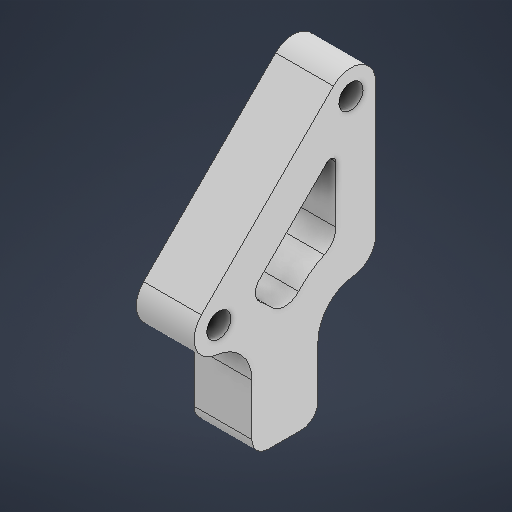
# Autodesk Inventor part: MOGO Mech
Saved by Autodesk Inventor 2025.1 (Build 291241000, 241)
## iProperties
Created: 2024-11-22
Part Number: MOGO Mech
Material: Generic
Document SubType Name: Modeling
Designer: Juanl
Density: 1 g/cm^3
Appearance: Default
Mass: 11.7203 g
Surface Area: 40.8724 cm^2
Volume: 11.7203 cm^3
Author: Juanl
Autodesk Inventor part; units mm, degrees
ref_plane "YZ Plane" through (0, 0, 0) normal (1, 0, 0) x (0, 1, 0)
ref_plane "XZ Plane" through (0, 0, 0) normal (0, 1, 0) x (-1, 0, 0)
ref_plane "XY Plane" through (0, 0, 0) normal (0, 0, 1) x (1, 0, 0)
sketch "Sketch1" plane through (0, 0, 0) normal (1, 0, 0) x (0, 1, 0)
  line L0 (-12.6683, 12.8416) -> (-12.6683, 0.1416)
  line L1 (-12.6683, 0.1416) -> (-12.6683, -12.5584)
  line L2 (-12.6683, -12.5584) -> (0.0318, -12.5584)
  line L3 (0.0318, -12.5584) -> (12.7318, -12.5584)
  circle A0 centre (-12.6683, 12.8416) radius 2.3241
  circle A1 centre (12.7318, -12.5584) radius 2.3241
  line L4 (-12.6683, 12.8416) -> (-12.6683, -12.5584) construction
  line L5 (-17.4308, 12.8416) -> (-17.4308, -12.5584)
  line L6 (-7.9058, -12.5584) -> (-7.9058, 12.8416)
  arc A2 (-7.9058, 12.8416) -> (-17.4308, 12.8416) centre (-12.6683, 12.8416) ccw
  arc A3 (-17.4308, -12.5584) -> (-7.9058, -12.5584) centre (-12.6683, -12.5584) ccw
  line L7 (12.7318, -12.5584) -> (-12.6683, -12.5584) construction
  line L8 (12.7318, -7.7959) -> (-12.6683, -7.7959)
  line L9 (-12.6683, -17.3209) -> (12.7318, -17.3209)
  arc A4 (12.7318, -17.3209) -> (12.7318, -7.7959) centre (12.7318, -12.5584) ccw
  arc A5 (-12.6683, -7.7959) -> (-12.6683, -17.3209) centre (-12.6683, -12.5584) ccw
  line L10 (-12.6683, 0.1416) -> (-38.0683, 0.1416)
  arc A6 (-7.9058, 4.3417) -> (-7.9058, -4.0585) centre (-12.6683, 0.1416) ccw
  line L11 (-12.6683, 6.4916) -> (-34.8933, 6.4916)
  line L12 (-38.0683, 3.3166) -> (-38.0683, -3.0334)
  line L13 (-34.8933, -6.2084) -> (-12.6683, -6.2084)
  arc A7 (-34.8933, 6.4916) -> (-38.0683, 3.3166) centre (-34.8933, 3.3166) ccw
  arc A8 (-38.0683, -3.0334) -> (-34.8933, -6.2084) centre (-34.8933, -3.0334) ccw
  point P0 (0, 0)
  point P1 (0.0317, -12.5584)
  point P2 (-7.9058, -7.7959)
  point P3 (-17.4308, -6.2084)
  point P4 (-17.4308, 6.4916)
  dimension "d1" = 4.6482
  dimension "d2" = 4.6482
  dimension "d3" = 9.525
  dimension "d7" = 25.4
  dimension "d8" = 12.7
  dimension "d9" = 3.175
  constraints: 32 end point, 16 point on circle, 13 tangent, 9 centre point, 5 point on line, 3 coincident, 3 perpendicular, 2 collinear, 2 parallel, 2 vertical, 1 concentric, 1 equal radius, 1 horizontal, 1 midpoint
  measures "d1" diameter of A0
  measures "d2" diameter of A1
  measures "d3" diameter of A3
  measures "d7" distance of L0.end L10.end
  measures "d8" diameter of A6
  measures "d9" radius of A7
extrude "Extrusion1" add sketch "Sketch1" along normal blind 11.1125
fillet "Fillet1" radius 7.62 1 edges at (5.5563, -17.4308, -6.2084)
sketch "Sketch3" plane through (11.1125, 0, 0) normal (1, 0, 0) x (0, 0, -1)
  arc A0 (-12.8416, -7.9058) -> (-12.8416, -17.4308) centre (-12.8416, -12.6683) ccw projected
  line L0 (-12.8416, -17.4308) -> (-6.4916, -17.4308) projected
  line L1 (-6.4916, -17.4308) -> (-6.4916, -34.8933) projected
  arc A1 (-6.4916, -34.8933) -> (-3.3166, -38.0683) centre (-3.3166, -34.8933) ccw projected
  line L2 (-3.3166, -38.0683) -> (3.0334, -38.0683) projected
  arc A2 (3.0334, -38.0683) -> (6.2084, -34.8933) centre (3.0334, -34.8933) ccw projected
  line L3 (6.2084, -34.8933) -> (6.2084, -24.9854) projected
  arc A3 (13.0468, -17.4056) -> (6.2084, -24.9854) centre (13.8284, -24.9854) ccw projected
  arc A4 (13.0468, -17.4056) -> (17.3209, -12.6683) centre (12.5584, -12.6683) ccw projected
  line L4 (17.3209, -12.6683) -> (17.3209, 12.7318) projected
  arc A5 (17.3209, 12.7318) -> (7.7959, 12.7318) centre (12.5584, 12.7318) ccw projected
  line L5 (7.7959, 12.7318) -> (7.7959, -7.9058) projected
  line L6 (7.7959, -7.9058) -> (-12.8416, -7.9058) projected
  circle A6 centre (-12.8416, -12.6683) radius 2.3241 projected
  circle A7 centre (12.5584, 12.7318) radius 2.3241 projected
  line L7 (-16.2092, -9.3007) -> (9.1908, 16.0993)
  arc A8 (-12.8416, -7.9058) -> (-12.8416, -17.4308) centre (-12.8416, -12.6683) ccw projected
  point P0 (0, 0)
  constraints: 2 end point, 2 point on circle, 2 tangent
extrude "Extrusion2" add sketch "Sketch3" against normal up to surface (11.1125 mm away) contours A0 L7 A5 L5 L6
fillet "Fillet2" radius 7.62 1 edges at (5.5563, -17.4308, 6.4916)
sketch "Sketch4" plane through (11.1125, 0, 0) normal (1, 0, 0) x (0, 0, -1)
  arc A0 (-16.2092, -9.3007) -> (-13.3301, -17.4056) centre (-12.8416, -12.6683) ccw projected
  arc A1 (-6.4916, -24.9854) -> (-13.3301, -17.4056) centre (-14.1116, -24.9854) ccw projected
  line L0 (-6.4916, -24.9854) -> (-6.4916, -34.8933) projected
  arc A2 (-6.4916, -34.8933) -> (-3.3166, -38.0683) centre (-3.3166, -34.8933) ccw projected
  line L1 (-3.3166, -38.0683) -> (3.0334, -38.0683) projected
  arc A3 (3.0334, -38.0683) -> (6.2084, -34.8933) centre (3.0334, -34.8933) ccw projected
  line L2 (6.2084, -34.8933) -> (6.2084, -24.9854) projected
  arc A4 (13.0468, -17.4056) -> (6.2084, -24.9854) centre (13.8284, -24.9854) ccw projected
  arc A5 (13.0468, -17.4056) -> (17.3209, -12.6683) centre (12.5584, -12.6683) ccw projected
  line L3 (17.3209, -12.6683) -> (17.3209, 12.7318) projected
  arc A6 (17.3209, 12.7318) -> (9.1908, 16.0993) centre (12.5584, 12.7318) ccw projected
  line L4 (9.1908, 16.0993) -> (-16.2092, -9.3007) projected
  circle A7 centre (-12.8416, -12.6683) radius 2.3241 projected
  circle A8 centre (12.5584, 12.7318) radius 2.3241 projected
  arc A9 (-0.1416, -18.7795) -> (-7.3449, -11.2783) centre (-14.1116, -24.9854) ccw
  arc A10 (9.6545, -10.2799) -> (-0.1416, -18.7795) centre (13.8284, -24.9854) ccw
  line L5 (9.6545, -10.2799) -> (9.6545, 5.7211)
  line L6 (9.6545, 5.7211) -> (-7.3449, -11.2783)
  point P0 (0, 0)
  constraints: 4 end point, 4 point on circle, 2 centre point, 3 other
extrude "Extrusion3" cut sketch "Sketch4" against normal blind 25.4 contours A9 L6 L5 A10
fillet "Fillet3" radius 3.81 1 edges at (5.5563, -10.2799, -9.6545)
fillet "Fillet4" radius 3.556 1 edges at (5.5563, -18.7795, 0.1416)
fillet "Fillet5" radius 2.54 1 edges at (5.5563, -11.2783, 7.3449)
fillet "Fillet6" radius 1.016 1 edges at (5.5563, 5.7211, -9.6545)
body "Solid1"
